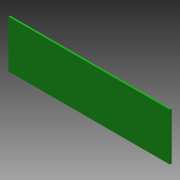
# Autodesk Inventor part: NavCom_PCB
Saved by Autodesk Inventor 2014 (Build 180170000, 170)
## iProperties
Created: 2017-02-12
Part Number: NavCom_PCB
Material: Všeobecné
Document SubType Name: Modeling
Designer: N
Density: 1 g/cm^3
Appearance: Výchozí
Author: N
Autodesk Inventor part; units mm, degrees
ref_plane "YZ Plane" through (0, 0, 0) normal (1, 0, 0) x (0, 1, 0)
ref_plane "XZ Plane" through (0, 0, 0) normal (0, 1, 0) x (-1, 0, 0)
ref_plane "XY Plane" through (0, 0, 0) normal (0, 0, 1) x (1, 0, 0)
sketch "Náčrt1" plane through (0, 0, 0) normal (0, 0, 1) x (1, 0, 0)
  line L0 (0, 0) -> (172.72, 0)
  line L1 (172.72, 0) -> (172.72, 50.8)
  line L2 (172.72, 50.8) -> (0, 50.8)
  line L3 (0, 50.8) -> (0, 0)
  constraints: 8 end point
extrude "Vysunutí1" add sketch "Náčrt1" along normal blind 1.905
